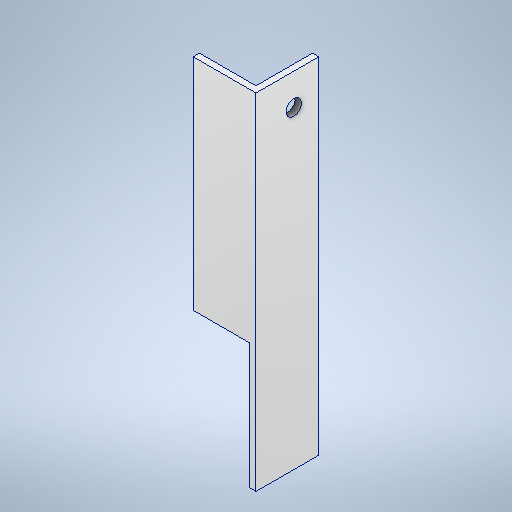
# Autodesk Inventor part: lift_tab
Saved by Autodesk Inventor 2025 (Build 290162000, 162)
## iProperties
Created: 2024-04-25
Part Number: lift_tab
Material: Hliník 6061
Document SubType Name: Modeling
Designer: rader
Density: 2.7 g/cm^3
Appearance: Hliník – plochý
Author: rader
Autodesk Inventor part; units mm, degrees
ref_plane "YZ Plane" through (0, 0, 0) normal (1, 0, 0) x (0, 1, 0)
ref_plane "XZ Plane" through (0, 0, 0) normal (0, 1, 0) x (-1, 0, 0)
ref_plane "XY Plane" through (0, 0, 0) normal (0, 0, 1) x (1, 0, 0)
sketch "Náčrt1" plane through (0, 0, 0) normal (0, 0, 1) x (1, 0, 0)
  line L0 (-12, 0) -> (2, 0) projected
  line L1 (0, 12) -> (0, -2) projected
  line L2 (0, 0) -> (0, 10)
  line L3 (0, 10) -> (-1, 10)
  line L4 (-1, 10) -> (-1, 1)
  line L5 (-1, 1) -> (-10, 1)
  line L6 (-10, 1) -> (-10, 0)
  line L7 (-10, 0) -> (0, 0)
  dimension "d0" = 10
  dimension "d1" = 1
  dimension "d2" = 9
  dimension "d3" = 9
  constraints: 12 end point, 3 perpendicular, 2 point on line, 1 collinear, 1 horizontal
  measures "d0" distance of L2.start L2.end
  measures "d1" distance of L2.end L3.end
  measures "d2" distance of L3.end L4.end
  measures "d3" distance of L4.end L5.end
extrude "Vysunutí1" add sketch "Náčrt1" along normal mid plane 55
sketch "Náčrt2" plane through (-1, 1, 27.5) normal (-1, 0, 0) x (0, 0, 1)
  line L0 (-55, 0) -> (0, 0) projected
  line L1 (0, 9) -> (0, 0) projected
  line L2 (-55, 9) -> (0, 9) projected
  line L3 (-55, 0) -> (-55, 9) projected
  point P0 (-27.5, -1)
  point P1 (-5, 5)
  dimension "d6" = 5
  dimension "d7" = 5
  measures "d6" distance from line of L1 point (-5, 5)
  measures "d7" distance from line of point (-5, 5) L0
hole "Díra1" at (-1, 6, 22.5) direction (1, 0, 0) diameter 2.459 end through all thread size "M3x0.5" class "6H" standard "ISO Metric profile"
sketch "Náčrt3" plane through (-10, 1, 27.5) normal (0, 1, 0) x (1, 0, 0)
  line L0 (0, 0) -> (0, 55) projected
  line L1 (9, 0) -> (0, 0) projected
  line L2 (9, 55) -> (9, 0) projected
  line L3 (0, 55) -> (9, 55) projected
  line L4 (0, 55) -> (9, 55)
  line L5 (9, 55) -> (9, 35)
  line L6 (9, 35) -> (0, 35)
  line L7 (0, 35) -> (0, 55)
  point P0 (10, 27.5)
  dimension "d15" = 20
  constraints: 8 end point, 2 parallel, 1 horizontal, 1 perpendicular, 1 point on line
  measures "d15" distance of L4.end L5.end
extrude "Vysunutí2" cut sketch "Náčrt3" against normal through all contours L0 L3 L2 L6
